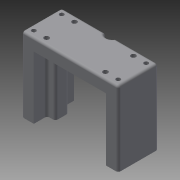
# Autodesk Inventor part: EncoderSupportOutside
Saved by Autodesk Inventor 2014 SP1 (Build 180222100, 222)
## iProperties
Created: 2015-03-28
Part Number: EncoderSupportOutside
Material: Generic
Document SubType Name: Modeling
Designer: david
Density: 1 g/cm^3
Appearance: Default
EncoderSupport_Space: 5,000 mm
EncoderSupportOutside_Length: 33,000 mm
EncoderSupportOutside_Width: 79,500 mm
Author: david
Autodesk Inventor part; units mm, degrees
ref_plane "YZ Plane" through (0, 0, 0) normal (1, 0, 0) x (0, 1, 0)
ref_plane "XZ Plane" through (0, 0, 0) normal (0, 1, 0) x (-1, 0, 0)
ref_plane "XY Plane" through (0, 0, 0) normal (0, 0, 1) x (1, 0, 0)
sketch "TopSketch" plane through (0, 0, 0) normal (0, 1, 0) x (-1, 0, 0)
  line L0 (-39.75, -16.5) -> (39.75, -16.5)
  line L1 (39.75, -16.5) -> (39.75, 16.5)
  line L2 (39.75, 16.5) -> (-39.75, 16.5)
  line L3 (-39.75, 16.5) -> (-39.75, -16.5)
  line L4 (-39.75, -16.5) -> (39.75, 16.5) construction
  line L5 (39.75, -16.5) -> (-39.75, 16.5) construction
  point P0 (0, 0)
  dimension "EncoderSupportOutside_Length" = 33
  dimension "EncoderSupportOutside_Width" = 79.5
  constraints: 12 end point, 2 midpoint, 2 parallel, 1 horizontal, 1 perpendicular
  measures "EncoderSupportOutside_Length" distance between parallel lines of L0 L2
  measures "EncoderSupportOutside_Width" distance between parallel lines of L1 L3
extrude "Top" add sketch "TopSketch" along normal blind 10
sketch "SideSketch" plane through (0, 0, 0) normal (0, -1, 0) x (1, 0, 0)
  line L0 (39.75, -16.5) -> (-39.75, -16.5) projected
  line L1 (39.75, 16.5) -> (39.75, -16.5) projected
  line L2 (-39.75, 16.5) -> (39.75, 16.5) projected
  line L3 (-39.75, -16.5) -> (-39.75, 16.5) projected
  line L4 (-29.75, 16.5) -> (-29.75, -16.5)
  line L5 (29.75, 16.5) -> (29.75, -16.5)
  line L6 (0, 0) -> (0, 21.6169) construction
  dimension "d4" = 10
  constraints: 6 end point, 4 point on line, 2 perpendicular, 1 parallel, 1 other
  measures "d4" distance between parallel lines of L3 L4
extrude "Side" add sketch "SideSketch" along normal blind 51.5 contours L0 L5 L2 L1 | L0 L3 L2 L4
sketch "CableHoleSketch" plane through (0, 10, 0) normal (0, 1, 0) x (1, 0, 0)
  line L0 (-39.75, -16.5) -> (39.75, -16.5) projected
  line L1 (39.75, -16.5) -> (39.75, 16.5) projected
  line L2 (0, 0) -> (0, 14.5107) construction
  circle A0 centre (0, 18.5) radius 4.75
  dimension "d7" = 9.5
  dimension "d8" = 35
  constraints: 2 end point, 1 centre point, 1 parallel, 1 point on line
  measures "d7" diameter of A0
  measures "d8" distance from line of L0 A0.centre
extrude "CableHole" cut sketch "CableHoleSketch" against normal up to next
sketch "InnerFixationHoleSketch" plane through (0, 10, 0) normal (0, 1, 0) x (1, 0, 0)
  line L0 (39.75, 16.5) -> (-39.75, 16.5) projected
  line L1 (39.75, 16.5) -> (-39.75, 16.5) projected
  circle A0 centre (-24.25, 11.5) radius 2
  line L2 (0, 0) -> (39.099, 0) construction
  line L3 (0, 0) -> (0, 35.9734) construction
  circle A1 centre (-24.25, -11.5) radius 2
  circle A2 centre (24.25, 11.5) radius 2
  circle A3 centre (24.25, -11.5) radius 2
  dimension "d11" = 4
  dimension "d12" = 5
  dimension "d13" = 24.25
  constraints: 4 centre point, 4 end point, 3 symmetric about line, 1 parallel, 1 perpendicular, 3 other
  measures "d11" diameter of A0
  measures "d12" distance from line of L0 A0.centre
  measures "d13" horizontal distance of L2.start A0.centre
extrude "InnerFixationHole" cut sketch "InnerFixationHoleSketch" against normal up to next
sketch "OuterFixationHoleSketch" plane through (0, 10, 0) normal (0, 1, 0) x (1, 0, 0)
  line L0 (39.75, 16.5) -> (-39.75, 16.5) projected
  line L1 (-39.75, 16.5) -> (-39.75, -16.5) projected
  line L2 (39.75, 16.5) -> (-39.75, 16.5) projected
  circle A0 centre (-34.75, 11.5) radius 1.75
  line L3 (0, 0) -> (36.9685, 0) construction
  line L4 (0, 0) -> (0, 24.5431) construction
  circle A1 centre (34.75, 11.5) radius 1.75
  circle A2 centre (-34.75, -11.5) radius 1.75
  circle A3 centre (34.75, -11.5) radius 1.75
  dimension "d16" = 3.5
  dimension "d17" = 5
  dimension "d18" = 5
  constraints: 4 centre point, 4 end point, 3 symmetric about line, 1 parallel, 1 perpendicular, 3 other
  measures "d16" diameter of A0
  measures "d17" distance from line of L1 A0.centre
  measures "d18" distance from line of L0 A0.centre
extrude "OuterFixationHole" cut sketch "OuterFixationHoleSketch" against normal up to next
sketch "CoilSpringHoleSketch" plane through (0, 0, 0) normal (0, -1, 0) x (1, 0, 0)
  circle A0 centre (24.25, -11.5) radius 2 projected
  circle A1 centre (-24.25, -11.5) radius 2 projected
  circle A2 centre (-24.25, 11.5) radius 2 projected
  circle A3 centre (24.25, 11.5) radius 2 projected
  line L0 (29.75, -16.5) -> (-29.75, -16.5) projected
  circle A4 centre (-24.25, 11.5) radius 3
  line L1 (0, 0) -> (0, 23.1959) construction
  line L2 (0, 0) -> (47.7515, 0) construction
  circle A5 centre (24.25, 11.5) radius 3
  circle A6 centre (-24.25, -11.5) radius 3
  circle A7 centre (24.25, -11.5) radius 3
  point P0 (-4.3084, -16.5)
  dimension "d21" = 6
  constraints: 4 centre point, 4 end point, 3 symmetric about line, 2 perpendicular, 1 coincident, 3 other
  measures "d21" diameter of A4
extrude "CoilSpringHole" cut sketch "CoilSpringHoleSketch" against normal blind 5
sketch "Sketch7" plane through (0, 0, 0) normal (0, -1, 0) x (1, 0, 0)
  circle A0 centre (-24.25, 11.5) radius 3 projected
  arc A1 (4.3084, -16.5) -> (-4.3084, -16.5) centre (0, -18.5) ccw projected
  line L0 (-29.75, 16.5) -> (-29.75, -16.5) projected
  line L1 (-29.75, 5.5) -> (-23, 5.5)
  line L2 (-23, 5.5) -> (-23, -5.5)
  line L3 (-23, -5.5) -> (-29.75, -5.5)
  line L4 (-29.75, -5.5) -> (-29.75, 5.5)
  line L5 (0, 0) -> (50.1862, 0) construction
  line L6 (0, 0) -> (0, -18.5) construction
  line L7 (29.75, 5.5) -> (23, 5.5)
  line L8 (23, 5.5) -> (23, -5.5)
  line L9 (23, -5.5) -> (29.75, -5.5)
  line L10 (29.75, -5.5) -> (29.75, 5.5)
  circle A2 centre (-24.25, 11.5) radius 3 construction
  dimension "d25" = 3
  dimension "d26" = 23
  constraints: 20 end point, 4 symmetric about line, 3 perpendicular, 2 parallel, 1 horizontal, 1 point on line, 1 other
  measures "d25" distance edge to line of A0 L1
  measures "d26" distance between parallel lines of L2 L6
extrude "Extrusion7" add sketch "Sketch7" along normal up to surface (51.5 mm away) contours L1 L2 L3 L0 | L10 L9 L8 L7
fillet "Fillet" radius 2 8 edges at (-29.75, -25.75, 5.5) (-23, -25.75, 5.5) (-23, -25.75, -5.5) (-29.75, -25.75, -5.5) (29.75, -25.75, 5.5) (23, -25.75, 5.5) (23, -25.75, -5.5) (29.75, -25.75, -5.5)
fillet "Fillet" radius 2 10 edges at (39.75, -20.75, -16.5) (-39.75, -20.75, -16.5) (22.0292, 10, -16.5) (0, 10, -13.75) (-22.0292, 10, -16.5) (39.75, 10, 0) (0, 10, 16.5) (-39.75, 10, 0) (-39.75, -20.75, 16.5) (39.75, -20.75, 16.5)
equation "\"EncoderSupportOutside_Length\" = EncoderSupportInside_Length"
equation "\"EncoderSupportOutside_Width\" = EncoderSupportInside_Width + 2 * EncoderSupportOutside_Thickness + 2 * EncoderSupportOutside_MecanicalSpace"
equation "\"d2\" = EncoderSupportOutside_Thickness"
equation "\"d4\" = EncoderSupportOutside_Thickness"
equation "\"d5\" = EncoderSupportInside_Height + EncoderSupport_Space"
equation "\"d7\" = Encoder_CableFixation_Diameter + EncoderSupport_PlasticShrinkingMargin"
equation "\"d8\" = Encoder_CableFixation_DistanceToTop + EncoderSupportInside_Front_Thickness"
equation "\"d9\" = EncoderSupportOutside_Thickness"
equation "\"d11\" = EncoderSupport_PlasticShrinkingMargin + EncoderSupport_FixationHole_Diameter + EncoderSupportOutside_MecanicalSpace"
equation "\"d12\" = EncoderSupport_FixationHole_Margin"
equation "\"d14\" = EncoderSupportOutside_Thickness"
equation "\"d16\" = EncoderSupport_FixationHole_Diameter + EncoderSupport_PlasticShrinkingMargin"
equation "\"d17\" = EncoderSupport_FixationHole_Margin"
equation "\"d18\" = EncoderSupport_FixationHole_Margin"
equation "\"d19\" = EncoderSupportOutside_Thickness"
equation "\"d21\" = EncoderSupport_CoilSpringHole_Diameter"
equation "\"d25\" = EncoderSupportInside_Hollow_Margin + EncoderSupportOutside_MecanicalSpace"
equation "\"d29\" = EncoderSupport_Fillet_Size"
equation "\"EncoderSupportOutside_Thickness\" = 10"
equation "\"EncoderSupportOutside_MecanicalSpace\" = 0.5"
equation "\"EncoderSupport_Space\" = 5"
equation "\"EncoderSupportInside_Length\" = 33"
equation "\"EncoderSupportInside_Width\" = 58.5"
equation "\"EncoderSupportInside_Height\" = 46.5"
equation "\"Encoder_CableFixation_Diameter\" = 9"
equation "\"EncoderSupport_PlasticShrinkingMargin\" = 0.5"
equation "\"Encoder_CableFixation_DistanceToTop\" = 32"
equation "\"EncoderSupportInside_Front_Thickness\" = 3"
equation "\"EncoderSupport_FixationHole_Diameter\" = 3"
equation "\"EncoderSupport_FixationHole_Margin\" = 5"
equation "\"EncoderSupport_CoilSpringHole_Diameter\" = 6"
equation "\"EncoderSupportInside_Hollow_Margin\" = 2.5"
equation "\"EncoderSupport_Fillet_Size\" = 2"
body "Solid1"
